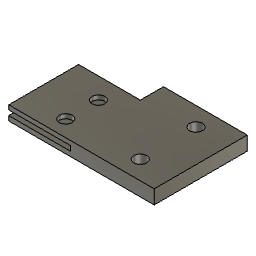
Schleppketten_Adapter_Y_bot (Autodesk Fusion 360 design; units mm, degrees)
Autodesk Fusion 360 part; units mm, degrees
sketch "Sketch1" plane through (0, 0, 0) normal (0, 0, 1) x (1, 0, 0)
  line L0 (0, 0) -> (26.5, 0)
  line L1 (26.5, 0) -> (26.5, 32)
  line L2 (26.5, 32) -> (0, 32)
  line L3 (0, 32) -> (0, 0)
  line L4 (0, 16) -> (26.5, 16) construction
  circle A0 centre (17.5, 23) radius 2.75
  circle A1 centre (17.5, 9) radius 2.75
  line L5 (17.5, 23) -> (17.5, 9) construction
  line L6 (14.75, 9) -> (17.5, 9) construction
  line L7 (26.5, 41.975) -> (62.5, 41.975)
  line L8 (62.5, 41.975) -> (62.5, 1.975)
  line L9 (62.5, 1.975) -> (26.5, 1.975)
  line L10 (26.5, 1.975) -> (26.5, 0)
  line L11 (48.5, 33.95) -> (48.5, 10) construction
  circle A2 centre (48.5, 33.95) radius 2.75
  circle A3 centre (48.5, 10) radius 2.75
  line L12 (62.5, 21.975) -> (48.5, 21.975) construction
  line L13 (26.5, 41.975) -> (26.5, 32)
  line L14 (0, 0) -> (0, 1.975)
  line L15 (0, 1.975) -> (26.5, 1.975)
  point P0 (14.75, 9)
  dimension "d1" = 26.5
  dimension "d3" = 14
  dimension "d7" = 40
  dimension "d8" = 22
  dimension "d9" = 5.5
  dimension "d10" = 14
  dimension "d12" = 23.95
  dimension "d13" = 17.5
  dimension "d14" = 5.5
  dimension "d20" = 9
  dimension "d22" = 1
  constraint horizontal L0
  constraint vertical L1
  constraint horizontal L2
  constraint vertical L3
  constraint coincident L0.start L3.end
  constraint midpoint L3 L4.start
  constraint coincident A0.centre L5.start
  constraint coincident A1.centre L5.end
  constraint perpendicular L4 L5
  constraint symmetric L4 A0.centre A1.centre
  constraint coincident A1 P0
  constraint coincident P0 L6.start
  constraint horizontal L6
  constraint equal A0 A1
  constraint coincident L1 L7.start
  constraint perpendicular L7 L8
  constraint coincident L0 L1.start
  constraint vertical L10
  constraint horizontal L9
  constraint perpendicular L2 L11
  constraint coincident L11.start A2.centre
  constraint coincident L11.end A3.centre
  constraint equal A2 A3
  constraint horizontal L7
  constraint midpoint L8 L12.start
  constraint midpoint L11 L12.end
  constraint horizontal L12
  constraint horizontal L4
  constraint coincident L1 L4.end
  constraint coincident L0.end L10
  constraint perpendicular L0 L14
  constraint horizontal L15
  measures "d1" distance of L0.start L0.end
  measures "d3" distance of A0.centre A1.centre
  measures "d7" distance of L7.end L8.end
  measures "d8" distance of L4.end L11
  measures "d9" diameter of A2
  measures "d10" horizontal distance of L8.end L11.end
  measures "d12" distance of L11.start L11.end
  measures "d13" horizontal distance of L0.start A1.centre
  measures "d14" diameter of A1
  measures "d20" vertical distance of L0.start A1.centre
  measures "d22" vertical distance of A1.centre L11.end
extrude "Extrude1" add sketch "Sketch1" along normal blind 6 contours L1 L2 L3 L15 | L1 L7 L8 L9 L13
extrude "Extrude2" cut sketch "Sketch1" along normal blind 2.1 from surface at 2 contours L0 L1 L3 L10 L14 L15 | L1 L2 L3 L15
equation "d3 = ( ( 9 + 19 ) / 2 ) * 1 mm"
equation "d12 = ( ( 17.5 + 30.4 ) / 2 ) * 1 mm"
equation "d15 = 2 mm + 2 mm + 2 mm"
